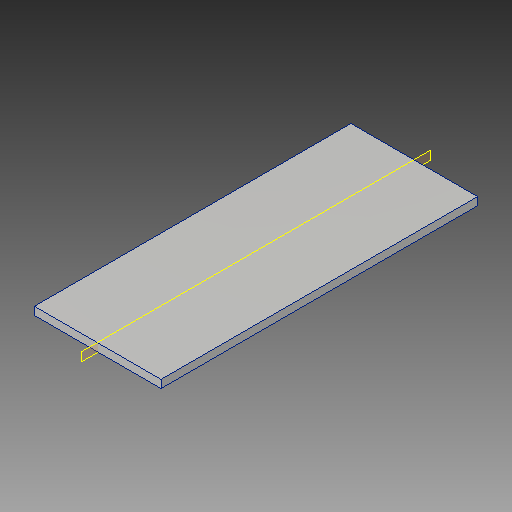
# Autodesk Inventor part: sheetPlateForBase
Saved by Autodesk Inventor 2017 (Build 210142000, 142)
## iProperties
Created: 2016-02-20
Part Number: sheetPlateForBase
Material: Aluminum 6061
Document SubType Name: Modeling
Designer: steele
Density: 2.7 g/cm^3
Appearance: Aluminum - Flat
Mass: 442.451 g
Surface Area: 561.289 cm^2
Volume: 163.871 cm^3
Author: steele
Autodesk Inventor part; units mm, degrees
ref_plane "XZ Plane" through (0, 0, 0) normal (0, 1, 0) x (-1, 0, 0)
ref_plane "XY Plane" through (0, 0, 0) normal (0, 0, 1) x (1, 0, 0)
sketch "Sketch1" plane through (0, 0, 0) normal (0, 1, 0) x (-1, 0, 0)
  line L0 (50.8, 127) -> (-50.8, 127)
  line L1 (-50.8, 127) -> (-50.8, -127)
  line L2 (-50.8, -127) -> (50.8, -127)
  line L3 (50.8, -127) -> (50.8, 127)
  line L4 (50.8, 127) -> (-50.8, -127) construction
  line L5 (-50.8, 127) -> (50.8, -127) construction
  point P0 (0, 0)
  dimension "d0" = 101.6
  dimension "d1" = 254
  constraints: 12 end point, 2 midpoint, 2 parallel, 1 horizontal, 1 perpendicular
  measures "d0" distance of L0.start L0.end
  measures "d1" distance of L2.end L0.start
extrude "Extrusion1" add sketch "Sketch1" along normal blind 6.35
equation "\"d0\" = width"
equation "\"d1\" = length"
equation "\"d2\" = materialThickness"
equation "\"width\" = 101.6"
equation "\"length\" = 254"
equation "\"materialThickness\" = 6.35"
body "Solid1"
